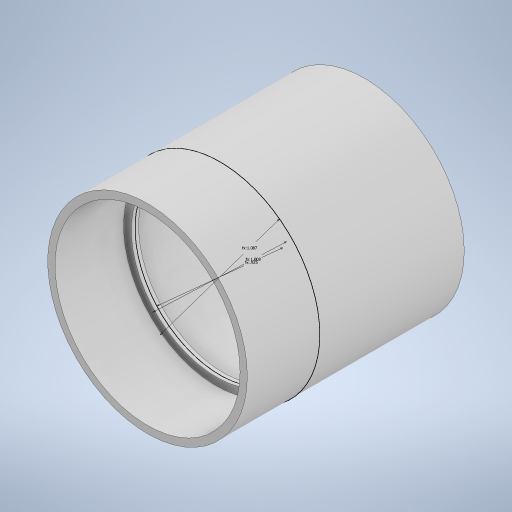
# Autodesk Inventor part: EimarFilterHolder
Saved by Autodesk Inventor 2024 (Build 280153000, 153)
## iProperties
Created: 2023-05-29
Part Number: EimarFilterHolder
Material: Generic
Document SubType Name: Modeling
Designer: Andrei
Density: 1 g/cm^3
Appearance: Default
Author: Andrei
Autodesk Inventor part; units mm, degrees
ref_plane "YZ Plane" through (0, 0, 0) normal (1, 0, 0) x (0, 1, 0)
ref_plane "XZ Plane" through (0, 0, 0) normal (0, 1, 0) x (-1, 0, 0)
ref_plane "XY Plane" through (0, 0, 0) normal (0, 0, 1) x (1, 0, 0)
sketch "Sketch1" plane through (0, 0, 0) normal (0, 0, 1) x (1, 0, 0)
  circle A0 centre (0, 0) radius 11.75
  circle A1 centre (0, 0) radius 12.8
  circle A2 centre (0, 0) radius 13.8
  dimension "d0" = 23.5
  dimension "d1" = 25.6
  dimension "d2" = 27.6
  constraints: 3 centre point, 3 coincident
  measures "d0" diameter of A0
  measures "d1" diameter of A1
  measures "d2" diameter of A2
extrude "Extrusion1" add sketch "Sketch1" along normal mid plane 1 contours A1
extrude "Extrusion2" add sketch "Sketch1" along normal blind 10 and the other way blind 20 contours A2
equation "\"d0\" = dInternal"
equation "\"d1\" = dFilter"
equation "\"d2\" = dFilter + wWall"
equation "\"d3\" = 0.5 * wCentral"
equation "\"d5\" = lFront"
equation "\"d6\" = lBack"
equation "\"wWall\" = 2"
equation "\"dFilter\" = 25.6"
equation "\"dInternal\" = 23.5"
equation "\"wCentral\" = 2"
equation "\"lFront\" = 10"
equation "\"lBack\" = 20"
body "Solid1"
